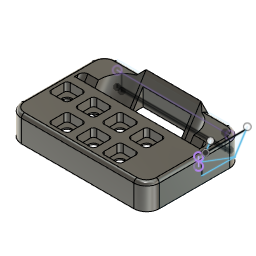
Base (Autodesk Fusion 360 design; units mm, degrees)
Autodesk Fusion 360 part; units mm, degrees
note: some values were not read from the file. Chosen so that the rebuilt part matches the saved one: which bodies a step acts on; which pieces of a blend or face edit are solid.
sketch "Sketch1" plane through (0, 0, 0) normal (0, 0, 1) x (1, 0, 0)
  line L0 (-34.5, 29) -> (51.5, 29)
  line L1 (83.5, -3) -> (-66.5, -3)
  line L2 (-83, -3) -> (100, -3)
  line L3 (107, -10) -> (107, -15)
  line L4 (107, -15) -> (-90, -15)
  line L5 (-90, -15) -> (-90, -10)
  line L6 (-85, -30) -> (-65, -30)
  line L7 (-60, -35) -> (-60, -55)
  line L8 (-65, -60) -> (-85, -60)
  line L9 (-90, -55) -> (-90, -35)
  circle A0 centre (-75, -45) radius 8
  circle A1 centre (-33.25, -45) radius 8
  line L10 (-18.25, -35) -> (-18.25, -55)
  line L11 (-48.25, -55) -> (-48.25, -35)
  line L12 (-23.25, -60) -> (-43.25, -60)
  line L13 (-43.25, -30) -> (-23.25, -30)
  circle A2 centre (8.5, -45) radius 8
  line L14 (23.5, -35) -> (23.5, -55)
  line L15 (-6.5, -55) -> (-6.5, -35)
  line L16 (18.5, -60) -> (-1.5, -60)
  line L17 (-1.5, -30) -> (18.5, -30)
  circle A3 centre (50.25, -45) radius 8
  line L18 (65.25, -35) -> (65.25, -55)
  line L19 (35.25, -55) -> (35.25, -35)
  line L20 (60.25, -60) -> (40.25, -60)
  line L21 (40.25, -30) -> (60.25, -30)
  circle A4 centre (-33.25, -86.75) radius 8
  line L22 (-18.25, -76.75) -> (-18.25, -96.75)
  line L23 (-48.25, -96.75) -> (-48.25, -76.75)
  line L24 (-23.25, -101.75) -> (-43.25, -101.75)
  line L25 (-43.25, -71.75) -> (-23.25, -71.75)
  circle A5 centre (8.5, -86.75) radius 8
  line L26 (23.5, -76.75) -> (23.5, -96.75)
  line L27 (-6.5, -96.75) -> (-6.5, -76.75)
  line L28 (18.5, -101.75) -> (-1.5, -101.75)
  line L29 (-1.5, -71.75) -> (18.5, -71.75)
  circle A6 centre (50.25, -86.75) radius 8
  line L30 (65.25, -76.75) -> (65.25, -96.75)
  line L31 (35.25, -96.75) -> (35.25, -76.75)
  line L32 (60.25, -101.75) -> (40.25, -101.75)
  line L33 (40.25, -71.75) -> (60.25, -71.75)
  arc A7 (-85, -30) -> (-90, -35) centre (-85, -35) ccw
  arc A8 (-60, -35) -> (-65, -30) centre (-65, -35) ccw
  arc A9 (-65, -60) -> (-60, -55) centre (-65, -55) ccw
  arc A10 (-90, -55) -> (-85, -60) centre (-85, -55) ccw
  arc A11 (-43.25, -30) -> (-48.25, -35) centre (-43.25, -35) ccw
  arc A12 (-18.25, -35) -> (-23.25, -30) centre (-23.25, -35) ccw
  arc A13 (-23.25, -60) -> (-18.25, -55) centre (-23.25, -55) ccw
  arc A14 (-48.25, -55) -> (-43.25, -60) centre (-43.25, -55) ccw
  arc A15 (-1.5, -30) -> (-6.5, -35) centre (-1.5, -35) ccw
  arc A16 (-6.5, -55) -> (-1.5, -60) centre (-1.5, -55) ccw
  arc A17 (18.5, -60) -> (23.5, -55) centre (18.5, -55) ccw
  arc A18 (23.5, -35) -> (18.5, -30) centre (18.5, -35) ccw
  arc A19 (40.25, -30) -> (35.25, -35) centre (40.25, -35) ccw
  arc A20 (65.25, -35) -> (60.25, -30) centre (60.25, -35) ccw
  arc A21 (60.25, -60) -> (65.25, -55) centre (60.25, -55) ccw
  arc A22 (35.25, -55) -> (40.25, -60) centre (40.25, -55) ccw
  arc A23 (40.25, -71.75) -> (35.25, -76.75) centre (40.25, -76.75) ccw
  arc A24 (65.25, -76.75) -> (60.25, -71.75) centre (60.25, -76.75) ccw
  arc A25 (60.25, -101.75) -> (65.25, -96.75) centre (60.25, -96.75) ccw
  arc A26 (35.25, -96.75) -> (40.25, -101.75) centre (40.25, -96.75) ccw
  arc A27 (18.5, -101.75) -> (23.5, -96.75) centre (18.5, -96.75) ccw
  arc A28 (23.5, -76.75) -> (18.5, -71.75) centre (18.5, -76.75) ccw
  arc A29 (-1.5, -71.75) -> (-6.5, -76.75) centre (-1.5, -76.75) ccw
  arc A30 (-6.5, -96.75) -> (-1.5, -101.75) centre (-1.5, -96.75) ccw
  arc A31 (-23.25, -101.75) -> (-18.25, -96.75) centre (-23.25, -96.75) ccw
  arc A32 (-48.25, -96.75) -> (-43.25, -101.75) centre (-43.25, -96.75) ccw
  arc A33 (-43.25, -71.75) -> (-48.25, -76.75) centre (-43.25, -76.75) ccw
  arc A34 (-18.25, -76.75) -> (-23.25, -71.75) centre (-23.25, -76.75) ccw
  arc A35 (-34.5, 29) -> (-66.5, -3) centre (-34.5, -3) ccw
  arc A36 (83.5, -3) -> (51.5, 29) centre (51.5, -3) ccw
  arc A37 (107, -10) -> (100, -3) centre (100, -10) ccw
  arc A38 (-83, -3) -> (-90, -10) centre (-83, -10) ccw
  line L34 (97, 39) -> (-80, 39)
  line L35 (-100, 19) -> (-100, -91.75)
  line L36 (-80, -111.75) -> (97, -111.75)
  line L37 (117, -91.75) -> (117, 19)
  arc A39 (-80, 39) -> (-100, 19) centre (-80, 19) ccw
  arc A40 (-100, -91.75) -> (-80, -111.75) centre (-80, -91.75) ccw
  arc A41 (117, 19) -> (97, 39) centre (97, 19) ccw
  arc A42 (97, -111.75) -> (117, -91.75) centre (97, -91.75) ccw
  line L38 (-34.5, 29) -> (51.5, 29)
  line L39 (-29.5, 29) -> (46.5, 29)
  point P0 (-90, -3)
  point P1 (107, -3)
  point P2 (-90, -30)
  point P3 (-60, -60)
  point P4 (-90, -60)
  dimension "d9" = 16
  dimension "d10" = 30
  dimension "d11" = 30
  dimension "d12" = 15
  dimension "d13" = 15
  dimension "d14" = 12
  dimension "d15" = 197
  dimension "d17" = 15
  dimension "d23" = 5
  dimension "d24" = 5
  dimension "d25" = 5
  dimension "d26" = 32
  dimension "d27" = 23.5
  dimension "d28" = 150
  dimension "d29" = 32
  dimension "d30" = 32
  dimension "d31" = 7
  dimension "d32" = 7
  dimension "d33" = 75
  dimension "d34" = 10
  dimension "d35" = 10
  dimension "d36" = 10
  dimension "d37" = 96.75
  dimension "d38" = 20
  dimension "d39" = 20
  dimension "d40" = 20
  dimension "d41" = 20
  dimension "d50" = 16
  dimension "d51" = 16
  dimension "d52" = 16
  dimension "d53" = 16
  dimension "d54" = 16
  dimension "d55" = 16
  constraint horizontal L0
  constraint horizontal L1
  constraint horizontal L2
  constraint vertical L3
  constraint horizontal L4
  constraint vertical L5
  constraint horizontal L6
  constraint horizontal L8
  constraint vertical L9
  constraint collinear L1 L2
  constraint coincident P2 L6
  constraint coincident P2 L9
  constraint tangent L6 A7
  constraint tangent L9 A7
  constraint tangent L6 A8
  constraint tangent L7 A8
  constraint coincident P3 L7
  constraint coincident P3 L8
  constraint tangent L7 A9
  constraint tangent L8 A9
  constraint equal A8 A9
  constraint coincident P4 L8
  constraint coincident P4 L9
  constraint tangent L8 A10
  constraint tangent L9 A10
  constraint equal A8 A10
  constraint tangent L11 A11
  constraint tangent L13 A11
  constraint tangent L10 A12
  constraint tangent L13 A12
  constraint equal A11 A12
  constraint tangent L10 A13
  constraint tangent L12 A13
  constraint equal A11 A13
  constraint tangent L11 A14
  constraint tangent L12 A14
  constraint equal A11 A14
  constraint tangent L15 A15
  constraint tangent L17 A15
  constraint equal A11 A15
  constraint tangent L15 A16
  constraint tangent L16 A16
  constraint equal A11 A16
  constraint tangent L14 A17
  constraint tangent L16 A17
  constraint equal A11 A17
  constraint tangent L14 A18
  constraint tangent L17 A18
  constraint equal A11 A18
  constraint tangent L19 A19
  constraint tangent L21 A19
  constraint equal A11 A19
  constraint tangent L18 A20
  constraint tangent L21 A20
  constraint equal A11 A20
  constraint tangent L18 A21
  constraint tangent L20 A21
  constraint equal A11 A21
  constraint tangent L19 A22
  constraint tangent L20 A22
  constraint equal A11 A22
  constraint tangent L31 A23
  constraint tangent L33 A23
  constraint equal A11 A23
  constraint tangent L30 A24
  constraint tangent L33 A24
  constraint equal A11 A24
  constraint tangent L30 A25
  constraint tangent L32 A25
  constraint equal A11 A25
  constraint tangent L31 A26
  constraint tangent L32 A26
  constraint equal A11 A26
  constraint tangent L26 A27
  constraint tangent L28 A27
  constraint equal A11 A27
  constraint tangent L26 A28
  constraint tangent L29 A28
  constraint equal A11 A28
  constraint tangent L27 A29
  constraint tangent L29 A29
  constraint equal A11 A29
  constraint tangent L27 A30
  constraint tangent L28 A30
  constraint equal A11 A30
  constraint tangent L22 A31
  constraint tangent L24 A31
  constraint equal A11 A31
  constraint tangent L23 A32
  constraint tangent L24 A32
  constraint equal A11 A32
  constraint tangent L23 A33
  constraint tangent L25 A33
  constraint equal A11 A33
  constraint tangent L22 A34
  constraint tangent L25 A34
  constraint equal A11 A34
  constraint tangent L0 A35
  constraint coincident L1.end A35.end
  constraint tangent L0 A36
  constraint coincident L1.start A36.start
  constraint coincident P1 L2
  constraint coincident P1 L3
  constraint tangent L2 A37
  constraint tangent L3 A37
  constraint coincident P0 L2
  constraint coincident P0 L5
  constraint tangent L2 A38
  constraint tangent L5 A38
  constraint horizontal L34
  constraint vertical L35
  constraint horizontal L36
  constraint vertical L37
  constraint tangent L34 A39
  constraint tangent L35 A39
  constraint tangent L35 A40
  constraint tangent L36 A40
  constraint tangent L34 A41
  constraint tangent L37 A41
  constraint tangent L36 A42
  constraint tangent L37 A42
  constraint horizontal L38
  constraint horizontal L39
  constraint coincident L38 L39.start
  measures "d9" diameter of A0
  measures "d10" distance of P3 P4
  measures "d11" distance of P2 P4
  measures "d12" horizontal distance of P4 A0.centre
  measures "d13" vertical distance of P4 A0.centre
  measures "d14" distance of P1 L3.end
  measures "d15" distance of P0 P1
  measures "d17" distance of L4 L6
  measures "d23" radius of A7
  measures "d24" radius of A8
  measures "d25" radius of A11
  measures "d26" radius of A35
  measures "d27" distance of L5 L1.end
  measures "d28" distance of L1.start L1.end
  measures "d29" radius of A36
  measures "d30" distance of L0 L2
  measures "d31" radius of A37
  measures "d32" radius of A38
  measures "d33" horizontal distance of A2.centre L1.end
  measures "d34" distance of L0 L34
  measures "d35" distance of L3.end L37
  measures "d36" distance of L4.end L35
  measures "d37" distance of L4 L36
  measures "d38" radius of A39 A5
  measures "d39" radius of A40
  measures "d40" radius of A41
  measures "d41" radius of A42
  measures "d50" diameter of A1
  measures "d51" diameter of A4
  measures "d52" diameter of A5
  measures "d53" diameter of A2
  measures "d54" diameter of A6
  measures "d55" diameter of A3
extrude "Extrude1" add sketch "Sketch1" along normal blind 2 contours L6 L7 L8 L9 A7 A8 A9 A10 | L10 L11 L12 L13 A11 A12 A13 A14 | L14 L15 L16 L17 A15 A16 A17 A18 | L18 L19 L20 L21 A19 A20 A21 A22 | L22 L23 L24 L25 A31 A32 A33 A34 | L26 L27 L28 L29 A27 A28 A29 A30 | L30 L31 L32 L33 A23 A24 A25 A26 | L34 L35 L36 L37 A39 A40 A41 A42 makes body 1
extrude "Extrude2" add sketch "Sketch1" along normal blind 10 contours L34 L35 L36 L37 A39 A40 A41 A42 bodies 1
extrude "Extrude3" add 1 faces at (96.4167, -53.9167, 10) along direction (0, 0, 1) blind 5 on bodies 1 bodies 1
extrude "Extrude4" add sketch "Sketch1" along normal blind 15 contours L0 L1 L2 A35 A36 L38 L39 | L1 L2 L3 L4 L5 A37 A38 bodies 1
extrude "Extrude5" add sketch "Sketch1" against normal blind 25 contours L0 L1 L2 A35 A36 L38 L39 | L1 L2 L3 L4 L5 A37 A38 | L34 L35 L36 L37 A39 A40 A41 A42 bodies 1
sketch "Sketch2" plane through (0, 39, 0) normal (0, 1, 0) x (-1, 0, 0)
  line L0 (80, -25) -> (80, 15)
  line L1 (80, 15) -> (-97, 15)
  line L2 (-97, 15) -> (-97, -25)
  line L3 (-97, -25) -> (80, -25)
  line L4 (-97, -20) -> (80, -20)
  line L5 (80, -20) -> (80, -23)
  line L6 (80, -23) -> (-97, -23)
  line L7 (-97, -23) -> (-97, -20)
  line L8 (-97, 0) -> (80, 0)
  line L9 (-90, 0) -> (73, 0)
  line L10 (73, 0) -> (73, -20)
  line L11 (73, -20) -> (-90, -20)
  line L12 (-90, -20) -> (-90, 0)
  line L13 (-90, -23) -> (73, -23)
  line L14 (73, -23) -> (73, -25)
  line L15 (73, -25) -> (-90, -25)
  line L16 (-90, -25) -> (-90, -23)
  dimension "d59" = 23
  dimension "d60" = 3
  dimension "d61" = 7
  dimension "d62" = 163
  dimension "d63" = 7
  dimension "d64" = 7
  constraint horizontal L4
  constraint vertical L5
  constraint horizontal L6
  constraint vertical L7
  constraint coincident L0 L5.end
  constraint coincident L2 L4.start
  constraint horizontal L9
  constraint vertical L10
  constraint horizontal L11
  constraint vertical L12
  constraint coincident L4 L10.end
  constraint coincident L8 L9.start
  constraint horizontal L13
  constraint vertical L14
  constraint horizontal L15
  constraint vertical L16
  constraint coincident L3 L14.end
  constraint coincident L6 L13.start
  measures "d59" distance of L6 L8
  measures "d60" distance of L4 L6
  measures "d61" distance of L7 L12
  measures "d62" distance of L10.end L11.end
  measures "d63" distance of L7 L16
  measures "d64" distance of L5 L14
extrude "Extrude6" cut sketch "Sketch2" against normal blind 85 from surface at -60 contours L4 L8 L9 L10 L11 L12 bodies 1
extrude "Extrude7" add sketch "Sketch1" against normal blind 7 from surface at -18 contours L6 L7 L8 L9 A7 A8 A9 A10 | A0 | A1 | L10 L11 L12 L13 A11 A12 A13 A14 | A2 | L14 L15 L16 L17 A15 A16 A17 A18 | A3 | L18 L19 L20 L21 A19 A20 A21 A22 | A4 | L22 L23 L24 L25 A31 A32 A33 A34 | A5 | L26 L27 L28 L29 A27 A28 A29 A30 | A6 | L30 L31 L32 L33 A23 A24 A25 A26 bodies 1
extrude "Extrude8" cut sketch "Sketch2" against normal up to surface (145 mm away) contours L0 L2 L4 L5 L6 L7 L11 L13 | L3 L6 L13 L14 L15 L16 bodies 1 makes body 2 at (55.25, -83.4167, -20) makes body 3 at (10.1667, -41.6667, -18) makes body 4 at (13.5, -83.4167, -18) makes body 5 at (48.5833, -41.6667, -18) makes body 6 at (-28.25, -48.3333, -18) makes body 7 at (5.1667, 16, 15)
chamfer "Chamfer1" distance 9 angle 45 1 edges at (-73, -30, -9) on bodies 7
sketch "Sketch3" plane through (117, 0, 0) normal (1, 0, 0) x (0, 1, 0)
  line L0 (19, -25) -> (19, 15)
  line L1 (19, 15) -> (-91.75, 15)
  line L2 (-91.75, 15) -> (-91.75, -25)
  line L3 (-91.75, -25) -> (19, -25)
  line L4 (-25, 5.6958) -> (26.8449, -13.702)
  line L5 (-25, 5.6958) -> (-25, -13.2374)
  line L6 (-25, -13.2374) -> (26.8449, -13.702)
  line L7 (26.8449, -13.702) -> (46.6838, 17.4228)
  line L8 (-25, 5.6958) -> (-11.1809, 27.3762)
  line L9 (-30, 2) -> (-30, 15)
  line L10 (-19.0695, 15) -> (45.1395, 15)
  dimension "d75" = 20
  dimension "d77" = 102
  dimension "d78" = 78
  dimension "d79" = 5
  constraint coincident L8 L10.start
  constraint coincident L1 L10.start
  constraint coincident L7 L10.end
  constraint parallel L1 L10
  measures "d75" angle of L4 L6
  measures "d77" angle of L4 L7
  measures "d78" angle of L4 L8
  measures "d79" distance of L5 L9
ref_plane "WorkPlane1" through (8.5, -15, 5) normal (0, -0.848048, 0.529919) x (-1, 0, 0)
sketch "Sketch4" plane through (0, -13.0348, 8.145) normal (0, -0.848048, 0.529919) x (-1, 0, 0)
  line L0 (130, -50) -> (-150, -50)
  constraint horizontal L0
ref_plane "WorkPlane2" through (10, 13.4612, 50.5474) normal (0, 0.529919, 0.848048) x (1, 0, 0)
sketch "Sketch5" plane through (0, 26.496, 42.4024) normal (0, 0.529919, 0.848048) x (1, 0, 0)
  line L0 (-34.5, 20.6098) -> (51.5, 20.6098)
  line L1 (83.5, -11.3902) -> (-66.5, -11.3902)
  line L2 (-83, -11.3902) -> (100, -11.3902)
  line L3 (107, -23.3902) -> (-90, -23.3902)
  arc A0 (83.5, -11.3902) -> (51.5, 20.6098) centre (51.5, -11.3902) ccw
  line L4 (107, -18.3902) -> (107, -23.3902)
  arc A1 (107, -18.3902) -> (100, -11.3902) centre (100, -18.3902) ccw
  line L5 (-90, -23.3902) -> (-90, -18.3902)
  arc A2 (-34.5, 20.6098) -> (-66.5, -11.3902) centre (-34.5, -11.3902) ccw
  arc A3 (-83, -11.3902) -> (-90, -18.3902) centre (-83, -18.3902) ccw
  line L6 (-43.25, -33.3902) -> (-23.25, -33.3902)
  point P0 (97, 19)
  point P1 (-80, 19)
  point P2 (-90, -11.3902)
  point P3 (107, -11.3902)
  dimension "d82" = 12
  dimension "d83" = 197
  dimension "d84" = 32
  dimension "d85" = 23.5
  dimension "d86" = 150
  dimension "d87" = 32
  dimension "d88" = 32
  dimension "d89" = 7
  dimension "d90" = 7
  dimension "d93" = 10
  constraint horizontal L0
  constraint horizontal L1
  constraint horizontal L2
  constraint vertical L4
  constraint horizontal L3
  constraint vertical L5
  constraint collinear L1 L2
  constraint tangent L0 A2
  constraint coincident L1.end A2.end
  constraint tangent L0 A0
  constraint coincident L1.start A0.start
  constraint coincident P3 L2
  constraint coincident P3 L4
  constraint tangent L2 A1
  constraint tangent L4 A1
  constraint coincident P2 L2
  constraint coincident P2 L5
  constraint tangent L2 A3
  constraint tangent L5 A3
  measures "d82" distance of L3.start P3
  measures "d83" distance of P2 P3
  measures "d84" radius of A2
  measures "d85" distance of L1.end L5
  measures "d86" distance of L1.end L1.start
  measures "d87" radius of A0
  measures "d88" distance of L0 L2
  measures "d89" radius of A1
  measures "d90" radius of A3
  measures "d93" distance of L3 L6
extrude "Extrude9" cut sketch "Sketch5" against normal blind 58 bodies 1 2 3 4 5 6 7
sketch "Sketch6" plane through (0, 0, 15) normal (0, 0, 1) x (-1, 0, 0)
  line L0 (83, 4.0581) -> (66.5, 4.0581)
  ellipse E0 centre (34.5, 4.0581) end of major axis (34.5, -33.6756) minor radius 32 (34.5, -33.6756) -> (66.5, 4.0581) ccw
  line L1 (34.5, -33.6756) -> (-51.5, -33.6756)
  ellipse E1 centre (-51.5, 4.0581) end of major axis (-51.5, 41.7918) minor radius 32 (-83.5, 4.0581) -> (-51.5, -33.6756) ccw
  line L2 (-83.5, 4.0581) -> (-100, 4.0581)
  ellipse E2 centre (-100, 12.3123) end of major axis (-100, 20.5666) minor radius 7 (-107, 12.3123) -> (-100, 4.0581) ccw
  line L3 (-107, 12.3123) -> (-107, 18.2082)
  line L4 (-107, 18.2082) -> (90, 18.2082)
  line L5 (90, 18.2082) -> (90, 12.3123)
  ellipse E3 centre (83, 12.3123) end of major axis (83, 4.0581) minor radius 7 (83, 4.0581) -> (90, 12.3123) ccw
  arc A0 (85, 30) -> (90, 35) centre (85, 35) ccw
  line L6 (85, 30) -> (65, 30)
  arc A1 (60, 35) -> (65, 30) centre (65, 35) ccw
  line L7 (60, 35) -> (60, 55)
  arc A2 (65, 60) -> (60, 55) centre (65, 55) ccw
  line L8 (65, 60) -> (85, 60)
  arc A3 (90, 55) -> (85, 60) centre (85, 55) ccw
  line L9 (90, 55) -> (90, 35)
  arc A4 (43.25, 30) -> (48.25, 35) centre (43.25, 35) ccw
  line L10 (43.25, 30) -> (23.25, 30)
  arc A5 (18.25, 35) -> (23.25, 30) centre (23.25, 35) ccw
  line L11 (18.25, 35) -> (18.25, 55)
  arc A6 (23.25, 60) -> (18.25, 55) centre (23.25, 55) ccw
  line L12 (23.25, 60) -> (43.25, 60)
  arc A7 (48.25, 55) -> (43.25, 60) centre (43.25, 55) ccw
  line L13 (48.25, 55) -> (48.25, 35)
  arc A8 (-18.5, 60) -> (-23.5, 55) centre (-18.5, 55) ccw
  line L14 (-18.5, 60) -> (1.5, 60)
  arc A9 (6.5, 55) -> (1.5, 60) centre (1.5, 55) ccw
  line L15 (6.5, 55) -> (6.5, 35)
  arc A10 (1.5, 30) -> (6.5, 35) centre (1.5, 35) ccw
  line L16 (1.5, 30) -> (-18.5, 30)
  arc A11 (-23.5, 35) -> (-18.5, 30) centre (-18.5, 35) ccw
  line L17 (-23.5, 35) -> (-23.5, 55)
  arc A12 (-40.25, 30) -> (-35.25, 35) centre (-40.25, 35) ccw
  line L18 (-40.25, 30) -> (-60.25, 30)
  arc A13 (-65.25, 35) -> (-60.25, 30) centre (-60.25, 35) ccw
  line L19 (-65.25, 35) -> (-65.25, 55)
  arc A14 (-60.25, 60) -> (-65.25, 55) centre (-60.25, 55) ccw
  line L20 (-60.25, 60) -> (-40.25, 60)
  arc A15 (-35.25, 55) -> (-40.25, 60) centre (-40.25, 55) ccw
  line L21 (-35.25, 55) -> (-35.25, 35)
  arc A16 (-40.25, 71.75) -> (-35.25, 76.75) centre (-40.25, 76.75) ccw
  line L22 (-40.25, 71.75) -> (-60.25, 71.75)
  arc A17 (-65.25, 76.75) -> (-60.25, 71.75) centre (-60.25, 76.75) ccw
  line L23 (-65.25, 76.75) -> (-65.25, 96.75)
  arc A18 (-60.25, 101.75) -> (-65.25, 96.75) centre (-60.25, 96.75) ccw
  line L24 (-60.25, 101.75) -> (-40.25, 101.75)
  arc A19 (-35.25, 96.75) -> (-40.25, 101.75) centre (-40.25, 96.75) ccw
  line L25 (-35.25, 96.75) -> (-35.25, 76.75)
  arc A20 (1.5, 71.75) -> (6.5, 76.75) centre (1.5, 76.75) ccw
  line L26 (1.5, 71.75) -> (-18.5, 71.75)
  arc A21 (-23.5, 76.75) -> (-18.5, 71.75) centre (-18.5, 76.75) ccw
  line L27 (-23.5, 76.75) -> (-23.5, 96.75)
  arc A22 (-18.5, 101.75) -> (-23.5, 96.75) centre (-18.5, 96.75) ccw
  line L28 (-18.5, 101.75) -> (1.5, 101.75)
  arc A23 (6.5, 96.75) -> (1.5, 101.75) centre (1.5, 96.75) ccw
  line L29 (6.5, 96.75) -> (6.5, 76.75)
  arc A24 (23.25, 101.75) -> (18.25, 96.75) centre (23.25, 96.75) ccw
  line L30 (23.25, 101.75) -> (43.25, 101.75)
  arc A25 (48.25, 96.75) -> (43.25, 101.75) centre (43.25, 96.75) ccw
  line L31 (48.25, 96.75) -> (48.25, 76.75)
  arc A26 (43.25, 71.75) -> (48.25, 76.75) centre (43.25, 76.75) ccw
  line L32 (43.25, 71.75) -> (23.25, 71.75)
  arc A27 (18.25, 76.75) -> (23.25, 71.75) centre (23.25, 76.75) ccw
  line L33 (18.25, 76.75) -> (18.25, 96.75)
  arc A28 (-97, 111.75) -> (-117, 91.75) centre (-97, 91.75) ccw
  line L34 (-117, 91.75) -> (-117, -19)
  arc A29 (-117, -19) -> (-97, -39) centre (-97, -19) ccw
  line L35 (-97, -39) -> (80, -39)
  arc A30 (80, -39) -> (100, -19) centre (80, -19) ccw
  line L36 (100, -19) -> (100, 91.75)
  arc A31 (100, 91.75) -> (80, 111.75) centre (80, 91.75) ccw
  line L37 (80, 111.75) -> (-97, 111.75)
  line L38 (-51.5, -33.6756) -> (34.5, -33.6756)
  line L39 (34.5, -33.6756) -> (34.5, -39)
  line L40 (34.5, -39) -> (-51.5, -39)
  line L41 (-51.5, -39) -> (-51.5, -33.6756)
  constraint horizontal L38
  constraint vertical L39
  constraint horizontal L40
  constraint vertical L41
  constraint coincident L35 L39.end
  constraint coincident L1.end L38.start
extrude "Extrude10" add sketch "Sketch6" along normal blind 16 contours L1 L35 L38 L39 L40 L41 bodies 7
extrude "Extrude11" cut sketch "Sketch5" against normal blind 30 bodies 1 2 3 4 5 6 7
chamfer "Chamfer2" distance 8.52 angle 45 2 edges at (51.5, 36.3378, 15) (-34.5, 36.3378, 15) on bodies 7
sketch "Sketch7" plane through (0, 0, 15) normal (0, 0, 1) x (-1, 0, 0)
  line L0 (43.02, -32.3136) -> (43.02, -39)
  line L1 (43.02, -39) -> (80, -39)
  arc A0 (80, -39) -> (100, -19) centre (80, -19) ccw
  line L2 (100, -19) -> (100, 91.75)
  arc A1 (100, 91.75) -> (80, 111.75) centre (80, 91.75) ccw
  line L3 (80, 111.75) -> (-97, 111.75)
  arc A2 (-97, 111.75) -> (-117, 91.75) centre (-97, 91.75) ccw
  line L4 (-117, 91.75) -> (-117, -19)
  arc A3 (-117, -19) -> (-97, -39) centre (-97, -19) ccw
  line L5 (-97, -39) -> (-60.02, -39)
  line L6 (-60.02, -39) -> (-60.02, -32.3136)
  ellipse E0 centre (-51.5, 4.0581) end of major axis (-51.5, 41.7918) minor radius 32 (-83.5, 4.0581) -> (-60.02, -32.3136) ccw
  line L7 (-83.5, 4.0581) -> (-100, 4.0581)
  ellipse E1 centre (-100, 12.3123) end of major axis (-100, 20.5666) minor radius 7 (-107, 12.3123) -> (-100, 4.0581) ccw
  line L8 (-107, 12.3123) -> (-107, 18.2082)
  line L9 (-107, 18.2082) -> (90, 18.2082)
  line L10 (90, 18.2082) -> (90, 12.3123)
  ellipse E2 centre (83, 12.3123) end of major axis (83, 4.0581) minor radius 7 (83, 4.0581) -> (90, 12.3123) ccw
  line L11 (83, 4.0581) -> (66.5, 4.0581)
  ellipse E3 centre (34.5, 4.0581) end of major axis (34.5, -33.6756) minor radius 32 (43.02, -32.3136) -> (66.5, 4.0581) ccw
  arc A4 (85, 30) -> (90, 35) centre (85, 35) ccw
  line L12 (85, 30) -> (65, 30)
  arc A5 (60, 35) -> (65, 30) centre (65, 35) ccw
  line L13 (60, 35) -> (60, 55)
  arc A6 (65, 60) -> (60, 55) centre (65, 55) ccw
  line L14 (65, 60) -> (85, 60)
  arc A7 (90, 55) -> (85, 60) centre (85, 55) ccw
  line L15 (90, 55) -> (90, 35)
  arc A8 (43.25, 30) -> (48.25, 35) centre (43.25, 35) ccw
  line L16 (43.25, 30) -> (23.25, 30)
  arc A9 (18.25, 35) -> (23.25, 30) centre (23.25, 35) ccw
  line L17 (18.25, 35) -> (18.25, 55)
  arc A10 (23.25, 60) -> (18.25, 55) centre (23.25, 55) ccw
  line L18 (23.25, 60) -> (43.25, 60)
  arc A11 (48.25, 55) -> (43.25, 60) centre (43.25, 55) ccw
  line L19 (48.25, 55) -> (48.25, 35)
  arc A12 (-18.5, 60) -> (-23.5, 55) centre (-18.5, 55) ccw
  line L20 (-18.5, 60) -> (1.5, 60)
  arc A13 (6.5, 55) -> (1.5, 60) centre (1.5, 55) ccw
  line L21 (6.5, 55) -> (6.5, 35)
  arc A14 (1.5, 30) -> (6.5, 35) centre (1.5, 35) ccw
  line L22 (1.5, 30) -> (-18.5, 30)
  arc A15 (-23.5, 35) -> (-18.5, 30) centre (-18.5, 35) ccw
  line L23 (-23.5, 35) -> (-23.5, 55)
  arc A16 (-40.25, 30) -> (-35.25, 35) centre (-40.25, 35) ccw
  line L24 (-40.25, 30) -> (-60.25, 30)
  arc A17 (-65.25, 35) -> (-60.25, 30) centre (-60.25, 35) ccw
  line L25 (-65.25, 35) -> (-65.25, 55)
  arc A18 (-60.25, 60) -> (-65.25, 55) centre (-60.25, 55) ccw
  line L26 (-60.25, 60) -> (-40.25, 60)
  arc A19 (-35.25, 55) -> (-40.25, 60) centre (-40.25, 55) ccw
  line L27 (-35.25, 55) -> (-35.25, 35)
  arc A20 (-40.25, 71.75) -> (-35.25, 76.75) centre (-40.25, 76.75) ccw
  line L28 (-40.25, 71.75) -> (-60.25, 71.75)
  arc A21 (-65.25, 76.75) -> (-60.25, 71.75) centre (-60.25, 76.75) ccw
  line L29 (-65.25, 76.75) -> (-65.25, 96.75)
  arc A22 (-60.25, 101.75) -> (-65.25, 96.75) centre (-60.25, 96.75) ccw
  line L30 (-60.25, 101.75) -> (-40.25, 101.75)
  arc A23 (-35.25, 96.75) -> (-40.25, 101.75) centre (-40.25, 96.75) ccw
  line L31 (-35.25, 96.75) -> (-35.25, 76.75)
  arc A24 (1.5, 71.75) -> (6.5, 76.75) centre (1.5, 76.75) ccw
  line L32 (1.5, 71.75) -> (-18.5, 71.75)
  arc A25 (-23.5, 76.75) -> (-18.5, 71.75) centre (-18.5, 76.75) ccw
  line L33 (-23.5, 76.75) -> (-23.5, 96.75)
  arc A26 (-18.5, 101.75) -> (-23.5, 96.75) centre (-18.5, 96.75) ccw
  line L34 (-18.5, 101.75) -> (1.5, 101.75)
  arc A27 (6.5, 96.75) -> (1.5, 101.75) centre (1.5, 96.75) ccw
  line L35 (6.5, 96.75) -> (6.5, 76.75)
  arc A28 (23.25, 101.75) -> (18.25, 96.75) centre (23.25, 96.75) ccw
  line L36 (23.25, 101.75) -> (43.25, 101.75)
  arc A29 (48.25, 96.75) -> (43.25, 101.75) centre (43.25, 96.75) ccw
  line L37 (48.25, 96.75) -> (48.25, 76.75)
  arc A30 (43.25, 71.75) -> (48.25, 76.75) centre (43.25, 76.75) ccw
  line L38 (43.25, 71.75) -> (23.25, 71.75)
  arc A31 (18.25, 76.75) -> (23.25, 71.75) centre (23.25, 76.75) ccw
  line L39 (18.25, 76.75) -> (18.25, 96.75)
  line L40 (29.5, -13.2) -> (-46.5, -13.2)
  line L41 (-46.5, -13.2) -> (-46.5, -29.2)
  line L42 (-46.5, -29.2) -> (29.5, -29.2)
  line L43 (29.5, -29.2) -> (29.5, -13.2)
  line L44 (-97, -39) -> (80, -39)
  line L45 (-51.5, -38.9995) -> (-51.5, -13.2387)
  line L46 (34.5, -38.9995) -> (34.5, -13.2387)
  dimension "d102" = 16
  dimension "d103" = 25.8
  dimension "d104" = 5
  dimension "d105" = 5
  constraint horizontal L40
  constraint vertical L41
  constraint horizontal L42
  constraint vertical L43
  measures "d102" distance of L40.start L42.end
  measures "d103" distance of L40 L44
  measures "d104" distance of L41 L45
  measures "d105" distance of L43 L46
extrude "Extrude12" cut sketch "Sketch7" against normal through all contours L40 L41 L42 L43 bodies 1 2 3 4 5 6 7
extrude "Extrude13" cut 1 faces at (35.6667, -21, -6.6667) along direction (0, -1, 0) up to surface (85 mm away) on bodies 7 bodies 1 2 3 4 5 6 7
extrude "Extrude14" cut 1 faces at (-4.1667, 13.2, -18.4545) along direction (0, -1, 0) up to surface (34.2 mm away) on bodies 7 bodies 7
extrude "Extrude15" add 1 faces at (21.1667, -9.6, -17.6817) along direction (0, 0, -1) blind 0.2 on bodies 7 bodies 7 1 2 3 4 5 6
chamfer "Chamfer3" distance 20 angle 32 1 edges at (8.5, -21, -17.8817) measured on face at (21.1667, -9.6, -17.8817) on bodies 7
fillet "Fillet1" radius 20 1 edges at (-29.5, -21, -12.6922) on bodies 7
fillet "Fillet2" radius 20 1 edges at (46.5, -21, -12.6922) on bodies 7
fillet "Fillet3" radius 5 9 edges at (-61.51, 39, 15) (-94.1421, 33.1421, 15) (-100, -36.375, 15) (-94.1421, -105.8921, 15) (8.5, -111.75, 15) (111.1421, -105.8921, 15) (117, -36.375, 15) (111.1421, 33.1421, 15) (78.51, 39, 15) on bodies 7
